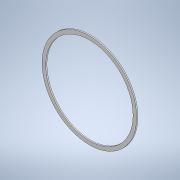
# Autodesk Inventor part: Прокладка клапана_CPY
Saved by Autodesk Inventor 2021 (Build 250183000, 183)
## iProperties
Created: 2020-11-15
Part Number: Прокладка клапана_CPY
Material: Типовые
Document SubType Name: Modeling
Designer: Тимоха
Density: 1 g/cm^3
Appearance: По умолчанию
Author: Тимоха
Autodesk Inventor part; units mm, degrees
ref_plane "YZ Plane" through (0, 0, 0) normal (1, 0, 0) x (0, 1, 0)
ref_plane "XZ Plane" through (0, 0, 0) normal (0, 1, 0) x (-1, 0, 0)
ref_plane "XY Plane" through (0, 0, 0) normal (0, 0, 1) x (1, 0, 0)
sketch "Эскиз1" plane through (0, 0, 0) normal (0, 0, 1) x (1, 0, 0)
  circle A0 centre (0, 0) radius 72.5
  circle A1 centre (0, 0) radius 78.5
  dimension "d0" = 145
  dimension "d1" = 157
  constraints: 2 centre point, 2 coincident
  measures "d0" diameter of A0
  measures "d1" diameter of A1
extrude "Выдавливание1" add sketch "Эскиз1" along normal blind 2
